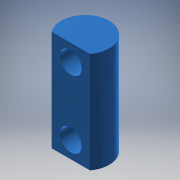
# Autodesk Inventor part: ExtruderQuickReleaseTensionDowel
Saved by Autodesk Inventor 2016 (Build 200138000, 138)
## iProperties
Category: Print
Created: 2015-05-04
Part Number: ExtruderQuickReleaseTensionDowel
Material: ABS Plastic
Document SubType Name: Modeling
Designer: Jack
Density: 1.06 g/cm^3
Appearance: Cyan
Vendor: Printed
Author: Jack
Title: Extruder Quick Release Tension Dowel
Autodesk Inventor part; units mm, degrees
ref_plane "YZ Plane" through (0, 0, 0) normal (1, 0, 0) x (0, 1, 0)
ref_plane "XZ Plane" through (0, 0, 0) normal (0, 1, 0) x (-1, 0, 0)
ref_plane "XY Plane" through (0, 0, 0) normal (0, 0, 1) x (1, 0, 0)
sketch "Sketch1" plane through (0, 0, 0) normal (0, 0, 1) x (1, 0, 0)
  arc A0 (4, -3) -> (-4, -3) centre (0, 0) ccw
  line L0 (-4, -3) -> (4, -3)
  dimension "d0" = 10
  dimension "d1" = 8
  constraints: 2 end point, 2 point on circle, 1 centre point, 1 coincident, 1 horizontal
  measures "d0" diameter of A0
  measures "d1" distance of L0.start L0.end
extrude "Extrusion1" add sketch "Sketch1" along normal blind 21
sketch "Sketch2" plane through (-4, -3, 0) normal (0, -1, 0) x (1, 0, 0)
  line L0 (8, 0) -> (0, 0) projected
  line L1 (8, 0) -> (8, 21) projected
  point P0 (4, 0)
  point P1 (4, 17.5)
  point P2 (4, 3.5)
  dimension "d6" = 4
  dimension "d14" = 14
  dimension "d15" = 3.5
  constraints: 1 vertical alignment
  measures "d6" distance from line of L1 point (4, 17.5)
  measures "d14" distance of point (4, 3.5) point (4, 17.5)
  measures "d15" distance from line of L0 point (4, 3.5)
hole "Hole1" at (0, -3, 17.5) at (0, -3, 3.5) direction (0, 1, 0) diameter 4.5 depth 8 tip angle 118
body "Solid1"
